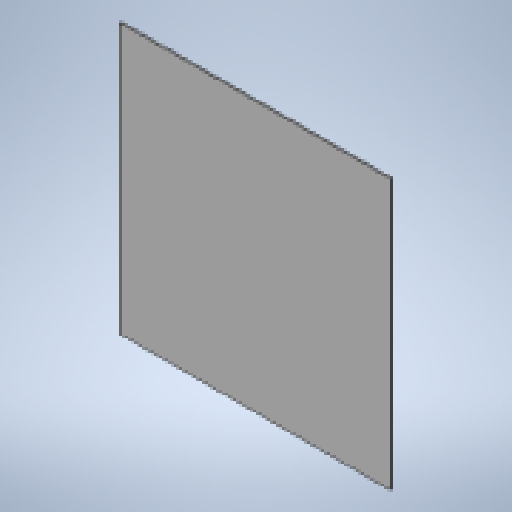
# Autodesk Inventor part: GBK 1111 shield 1_Dummy
Saved by Autodesk Inventor 2026.2 (Build 302298010, 298A)
## iProperties
Created: 2026-04-17
Part Number: GBK 1111 shield 1_Dummy
Material: Steel
Document SubType Name: Sheet Metal
Designer: admin
Stock Number: 1115
Mass: 69243.3 g
Surface Area: 44341.6 cm^2
Volume: 8820.8 cm^3
Density: 7.85 g/cm^3
Flat Pattern Width: 70 cm
Flat Pattern Length: 80 cm
Flat Pattern Area: 5600 cm^2
Sheet Metal Rule: Default_mm
Sheet Metal Width: 700,000 mm
Sheet Metal Length: 800,000 mm
Sheet Metal Area: 560000,000 mm^2
Appearance: Default
Author: admin
Autodesk Inventor part; units mm, degrees
ref_plane "YZ Plane" through (0, 0, 0) normal (1, 0, 0) x (0, 1, 0)
ref_plane "XZ Plane" through (0, 0, 0) normal (0, 1, 0) x (-1, 0, 0)
ref_plane "XY Plane" through (0, 0, 0) normal (0, 0, 1) x (1, 0, 0)
sketch "Sketch1" plane through (0, 0, 0) normal (0, 0, 1) x (1, 0, 0)
  line L0 (350, -400) -> (-350, -400)
  line L1 (-350, -400) -> (-350, 400)
  line L2 (-350, 400) -> (350, 400)
  line L3 (350, 400) -> (350, -400)
  line L4 (350, -400) -> (-350, 400) construction
  line L5 (-350, -400) -> (350, 400) construction
  point P0 (0, 0)
  dimension "d0" = 700
  dimension "d1" = 800
  measures "d0" distance of L1.end L2.end
  measures "d1" distance of L0.end L1.end
extrude "Plate1" add sketch "Sketch1" along normal blind 4
sketch "Sketch3" plane through (0, 0, 0) normal (0, 0, -1) x (-1, 0, 0)
  line L0 (-738.6395, 5.6667) -> (-680, 5.6667) projected
  line L1 (206.0719, 366.8104) -> (206.0719, 4.8587) construction
  line L2 (206.0719, 4.8587) -> (120.9163, 4.8587) construction
  line L3 (120.9163, 4.8587) -> (120.9163, 366.8104) construction
  line L4 (120.9163, 366.8104) -> (206.0719, 366.8104) construction
  ellipse E0 centre (299.5394, 398) end of major axis (299.5394, 428) minor radius 0.3401 (299.5394, 368) -> (299.8795, 398) ccw projected
  line L5 (299.5394, 368) -> (295.5396, 368) projected
  line L6 (319.9499, 156.8333) -> (350.29, 156.8333) projected
  line L7 (319.9499, 156.8333) -> (319.9499, 160.8333) projected
  line L8 (319.9499, -339.8333) -> (350.29, -339.8333) projected
  line L9 (319.9499, -339.8333) -> (319.9499, -335.8333) projected
  line L10 (295.5396, -400) -> (295.5396, -343.3333) projected
  line L11 (-204.4962, -400) -> (-204.4962, -343.3333) projected
  line L12 (-349.3197, -339.8333) -> (-290, -339.8333) projected
  line L13 (-290, -339.8333) -> (-290, -335.8333) projected
  line L14 (-349.3197, 156.8333) -> (-290, 156.8333) projected
  line L15 (-290, 156.8333) -> (-290, 160.8333) projected
  ellipse E1 centre (-200.4965, 398) end of major axis (-200.4965, 428) minor radius 0.3401 (-200.4965, 368) -> (-200.1564, 398) ccw projected
  line L16 (-200.4965, 368) -> (-204.4962, 368) projected
  point P0 (0, 0)
  constraints: 5 other
mark "Mark2"
equation "\"d2\" = Thickness"
equation "\"BendRadius\" = Thickness"
equation "\"BendReliefWidth\" = Thickness"
equation "\"BendReliefDepth\" = 0.5 * Thickness"
equation "\"CornerReliefSize\" = 4 * Thickness"
equation "\"MinimumRemnant\" = 2 * Thickness"
equation "\"TransitionRadius\" = BendRadius"
equation "\"JacobiRadiusSize\" = BendRadius"
equation "\"GapSize\" = Thickness"
equation "\"Thickness\" = 4"
body "Solid1"
